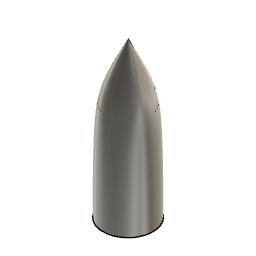
Nosce cone 1 v2 (Autodesk Fusion 360 design; units mm, degrees)
Autodesk Fusion 360 part; units mm, degrees
sketch "Sketch1" plane through (0, 0, 0) normal (1, 0, 0) x (0, 1, 0)
  line L0 (0, 0) -> (0, 279.4)
  line L1 (0, 0) -> (45.085, 0)
  spline S0 degree 2 poles (45.085, 0) (45.085, 191.8078) (0, 279.4) knots 0 0 0 28.694586 28.694586 28.694586 weights 1 3 1
  dimension "d1" = 279.4
  dimension "d2" = 45.085
  constraint coincident L0.start L1.start
  constraint vertical L0
  constraint perpendicular L0 L1
  measures "d1" distance of L0.start L0.end
  measures "d2" distance of L0.start L1.end
revolve "Revolve1" add sketch "Sketch1" angle 360 about axis through (0, 0, 0) along (0, 0, 1)
hole "Hole1" at (0, 0, 0) direction (0, 0, 1) diameter 76.2 depth 177.8 tip angle 118
hole "Hole2" at (0.6458, 7.381, 196.2409) direction (0.044889, 0.513078, 0.857167) diameter 50.8 depth 12.7 tip angle 118
equation "d2 = ( 3.55 / 2 ) * 1 in"
